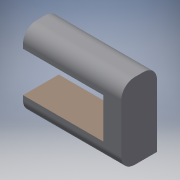
# Autodesk Inventor part: chamber_conn_holder
Saved by Autodesk Inventor 2016 (Build 200138000, 138)
## iProperties
Created: 2016-08-11
Part Number: chamber_conn_holder
Material: Generic
Document SubType Name: Modeling
Designer: GentnerLab
Density: 1 g/cm^3
Appearance: Default
Author: GentnerLab
Autodesk Inventor part; units mm, degrees
ref_plane "YZ Plane" through (0, 0, 0) normal (1, 0, 0) x (0, 1, 0)
ref_plane "XZ Plane" through (0, 0, 0) normal (0, 1, 0) x (-1, 0, 0)
ref_plane "XY Plane" through (0, 0, 0) normal (0, 0, 1) x (1, 0, 0)
sketch "Sketch1" plane through (0, 0, 0) normal (0, 1, 0) x (-1, 0, 0)
  line L0 (0, 0) -> (4.5, 0)
  line L1 (4.5, -2.25) -> (0, -2.25)
  line L2 (0, -2.25) -> (0, 0)
  dimension "d0" = 2.25
  constraints: 6 end point, 1 horizontal, 1 parallel
  measures "d0" distance between parallel lines of L1 L0
surface extrude "ExtrusionSrf1" sketch "Sketch1" along normal blind 2 shown yes curves L1 L2 L0
thicken "Thicken1" operation new thickness 1 both sides no extend neighbours no toward (1, 0, 0) faces at (0, 0.6667, -1.5) (-1.5, 0.6667, 0) (-3, 0.6667, -2.25)
fillet "Fillet1" radius 0.75 3 edges at (-1.75, 0, -3.25) (-1.75, 0, 1) (-1.75, 2, 1)
body "Solid1"
body "Srf1"
